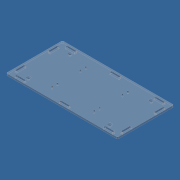
# Autodesk Inventor part: P1704_205
Saved by Autodesk Inventor 2015 (Build 190159000, 159)
## iProperties
Created: 2017-02-08
Part Number: P1704_205
Project: Manette
Material: Plastique PMMA
Description: Socle- Table
Document SubType Name: Modeling
Designer: Alexandre.PICOTTE
Authority: 185x93.4x3
Density: 1.188 g/cm^3
Appearance: Transparent - Clair
Mass: 59.5295 g
Surface Area: 366.091 cm^2
Volume: 50.109 cm^3
Material number: ---
Author: Boris.GAUDARD
Autodesk Inventor part; units mm, degrees
ref_plane "Plan YZ" through (0, 0, 0) normal (1, 0, 0) x (0, 1, 0)
ref_plane "Plan XZ" through (0, 0, 0) normal (0, 1, 0) x (-1, 0, 0)
ref_plane "Plan XY" through (0, 0, 0) normal (0, 0, 1) x (1, 0, 0)
sketch "Esquisse1" plane through (0, 0, 0) normal (0, 0, 1) x (1, 0, 0)
  line L0 (-92.5, 46.7) -> (92.5, 46.7)
  line L1 (92.5, 46.7) -> (92.5, -46.7)
  line L2 (92.5, -46.7) -> (-92.5, -46.7)
  line L3 (-92.5, -46.7) -> (-92.5, 46.7)
  line L4 (0, -65.38) -> (0, 65.38) construction
  line L5 (-129.5, 0) -> (129.5, 0) construction
  point P0 (0, 0)
  dimension "d0" = 185
  dimension "d1" = 93.4
  constraints: 8 end point, 2 parallel, 1 horizontal, 1 perpendicular, 2 other
  measures "d0" distance between parallel lines of L1 L3
  measures "d1" distance between parallel lines of L0 L2
extrude "Extrusion1" add sketch "Esquisse1" along normal blind 3
fillet "Congé1" radius 2 4 edges at (-92.5, 46.7, 1.5) (92.5, 46.7, 1.5) (92.5, -46.7, 1.5) (-92.5, -46.7, 1.5)
sketch "Esquisse21" plane through (0, 0, 3) normal (0, 0, 1) x (1, 0, 0)
  line L0 (-129.5, 0) -> (129.5, 0) construction
  line L1 (0, -85.38) -> (0, 87.38) construction
  line L2 (-7.5, 43.7) -> (7.5, 43.7)
  line L3 (7.5, 43.7) -> (7.5, 40.5)
  line L4 (7.5, 40.5) -> (-7.5, 40.5)
  line L5 (-7.5, 40.5) -> (-7.5, 43.7)
  line L6 (-90.5, 46.7) -> (90.5, 46.7) construction
  line L7 (-81, 43.7) -> (-66, 43.7)
  line L8 (-66, 43.7) -> (-66, 40.5)
  line L9 (-66, 40.5) -> (-81, 40.5)
  line L10 (-81, 40.5) -> (-81, 43.7)
  line L11 (-92.5, -44.7) -> (-92.5, 44.7) construction
  line L12 (66, 43.7) -> (81, 43.7)
  line L13 (81, 43.7) -> (81, 40.5)
  line L14 (81, 40.5) -> (66, 40.5)
  line L15 (66, 40.5) -> (66, 43.7)
  line L16 (-81, -40.5) -> (-66, -40.5)
  line L17 (-66, -40.5) -> (-66, -43.7)
  line L18 (-66, -43.7) -> (-81, -43.7)
  line L19 (-81, -43.7) -> (-81, -40.5)
  line L20 (-7.5, -43.7) -> (7.5, -43.7)
  line L21 (7.5, -43.7) -> (7.5, -40.5)
  line L22 (7.5, -40.5) -> (-7.5, -40.5)
  line L23 (-7.5, -40.5) -> (-7.5, -43.7)
  line L24 (66, -43.7) -> (81, -43.7)
  line L25 (81, -43.7) -> (81, -40.5)
  line L26 (81, -40.5) -> (66, -40.5)
  line L27 (66, -40.5) -> (66, -43.7)
  point P0 (0, 0)
  dimension "d216" = 15
  dimension "d217" = 3.2
  dimension "d218" = 3
  dimension "d221" = 11.5
  constraints: 48 end point, 12 parallel, 8 collinear, 6 horizontal, 6 perpendicular, 4 equal length, 1 point on line, 7 other
  measures "d216" distance of L2.start L2.end
  measures "d217" distance of L2.end L3.end
  measures "d218" distance between parallel lines of L6 L2
  measures "d221" distance between parallel lines of L10 L11
extrude "Extrusion8" cut sketch "Esquisse21" against normal through all
sketch "Esquisse23" plane through (0, 0, 3) normal (0, 0, 1) x (1, 0, 0)
  line L0 (0, -65.38) -> (0, 65.38) construction
  line L1 (-129.5, 0) -> (129.5, 0) construction
  point P0 (0, 0)
  point P1 (-67.5, 34.5)
  point P2 (67.5, 34.5)
  point P3 (67.5, -34.5)
  point P4 (-67.5, -34.5)
  dimension "d238" = 135
  dimension "d239" = 69
  constraints: 2 horizontal alignment, 2 symmetric about line, 2 vertical alignment
  measures "d238" distance of point (67.5, 34.5) point (-67.5, 34.5)
  measures "d239" distance of point (-67.5, -34.5) point (-67.5, 34.5)
hole "Perçage11" at (-67.5, 34.5, 3) at (67.5, 34.5, 3) at (67.5, -34.5, 3) at (-67.5, -34.5, 3) direction (0, 0, -1) diameter 3.4 end through all countersink diameter 6.3 countersink angle 90 clearance for "Vis à tête plate fraisée ISO 2009/7046" size "M3" standard "ISO"
sketch "Esquisse24" plane through (0, 0, 3) normal (0, 0, 1) x (1, 0, 0)
  line L0 (0, -87.38) -> (0, 85.38) construction
  line L1 (-89.5, 35.2) -> (-86.5, 35.2)
  line L2 (-86.5, 35.2) -> (-86.5, 20.2)
  line L3 (-86.5, 20.2) -> (-89.5, 20.2)
  line L4 (-89.5, 20.2) -> (-89.5, 35.2)
  line L5 (-89.5, -20.2) -> (-86.5, -20.2)
  line L6 (-86.5, -20.2) -> (-86.5, -35.2)
  line L7 (-86.5, -35.2) -> (-89.5, -35.2)
  line L8 (-89.5, -35.2) -> (-89.5, -20.2)
  line L9 (89.5, -35.2) -> (86.5, -35.2)
  line L10 (86.5, -35.2) -> (86.5, -20.2)
  line L11 (86.5, -20.2) -> (89.5, -20.2)
  line L12 (89.5, -20.2) -> (89.5, -35.2)
  line L13 (86.5, 35.2) -> (89.5, 35.2)
  line L14 (89.5, 35.2) -> (89.5, 20.2)
  line L15 (89.5, 20.2) -> (86.5, 20.2)
  line L16 (86.5, 20.2) -> (86.5, 35.2)
  line L17 (-92.5, -44.7) -> (-92.5, 44.7) construction
  line L18 (-129.5, 0) -> (129.5, 0) construction
  line L19 (90.5, -46.7) -> (-90.5, -46.7) construction
  point P0 (0, 0)
  dimension "d248" = 15
  dimension "d249" = 3
  dimension "d250" = 3
  dimension "d251" = 11.5
  constraints: 32 end point, 8 parallel, 4 collinear, 4 horizontal, 4 perpendicular, 3 point on line, 6 other
  measures "d248" distance of L7.end L5.start
  measures "d249" distance of L5.start L5.end
  measures "d250" distance between parallel lines of L17 L8
  measures "d251" distance between parallel lines of L7 L19
extrude "Extrusion10" cut sketch "Esquisse24" against normal through all
sketch "Esquisse26" plane through (0, 0, 3) normal (0, 0, 1) x (1, 0, 0)
  line L0 (-89.5, 35.2) -> (-86.5, 35.2) construction
  line L1 (-89.5, 20.2) -> (-89.5, 35.2) construction
  line L2 (-86.5, 35.2) -> (-86.5, 20.2) construction
  line L3 (-86.5, 20.2) -> (-89.5, 20.2) construction
  line L4 (-66, 40.5) -> (-81, 40.5) construction
  line L5 (-81, 40.5) -> (-81, 43.7) construction
  line L6 (-81, 43.7) -> (-66, 43.7) construction
  line L7 (-66, 43.7) -> (-66, 40.5) construction
  line L8 (7.5, 40.5) -> (-7.5, 40.5) construction
  line L9 (-7.5, 40.5) -> (-7.5, 43.7) construction
  line L10 (-7.5, 43.7) -> (7.5, 43.7) construction
  line L11 (7.5, 43.7) -> (7.5, 40.5) construction
  line L12 (81, 40.5) -> (66, 40.5) construction
  line L13 (66, 40.5) -> (66, 43.7) construction
  line L14 (66, 43.7) -> (81, 43.7) construction
  line L15 (81, 43.7) -> (81, 40.5) construction
  line L16 (-89.5, -35.2) -> (-89.5, -20.2) construction
  line L17 (-89.5, -20.2) -> (-86.5, -20.2) construction
  line L18 (-86.5, -20.2) -> (-86.5, -35.2) construction
  line L19 (-86.5, -35.2) -> (-89.5, -35.2) construction
  line L20 (-81, -40.5) -> (-66, -40.5) construction
  line L21 (-81, -43.7) -> (-81, -40.5) construction
  line L22 (-66, -43.7) -> (-81, -43.7) construction
  line L23 (-66, -40.5) -> (-66, -43.7) construction
  line L24 (89.5, -20.2) -> (89.5, -35.2) construction
  line L25 (89.5, -35.2) -> (86.5, -35.2) construction
  line L26 (86.5, -35.2) -> (86.5, -20.2) construction
  line L27 (86.5, -20.2) -> (89.5, -20.2) construction
  line L28 (-89.5, 20.2) -> (-89.5, 35.2) construction
  line L29 (-89.5, 35.2) -> (-86.5, 35.2) construction
  line L30 (-86.5, 35.2) -> (-86.5, 20.2) construction
  line L31 (-86.5, 20.2) -> (-89.5, 20.2) construction
  line L32 (-89.5, -35.2) -> (-89.5, -20.2) construction
  line L33 (-89.5, -20.2) -> (-86.5, -20.2) construction
  line L34 (-86.5, -20.2) -> (-86.5, -35.2) construction
  line L35 (-86.5, -35.2) -> (-89.5, -35.2) construction
  line L36 (86.5, 20.2) -> (86.5, 35.2) construction
  line L37 (86.5, 35.2) -> (89.5, 35.2) construction
  line L38 (89.5, 35.2) -> (89.5, 20.2) construction
  line L39 (89.5, 20.2) -> (86.5, 20.2) construction
  circle A0 centre (67.5, -34.5) radius 3.15 construction
  circle A1 centre (-67.5, 34.5) radius 3.15 construction
  circle A2 centre (67.5, 34.5) radius 3.15 construction
  circle A3 centre (-67.5, -34.5) radius 3.15 construction
  line L40 (7.5, -40.5) -> (7.5, -43.7) construction
  line L41 (7.5, -43.7) -> (-7.5, -43.7) construction
  line L42 (-7.5, -43.7) -> (-7.5, -40.5) construction
  line L43 (-7.5, -40.5) -> (7.5, -40.5) construction
  line L44 (66, 40.5) -> (66, 43.7) construction
  line L45 (66, 43.7) -> (81, 43.7) construction
  line L46 (81, 43.7) -> (81, 40.5) construction
  line L47 (81, 40.5) -> (66, 40.5) construction
  line L48 (-7.5, 40.5) -> (-7.5, 43.7) construction
  line L49 (-7.5, 43.7) -> (7.5, 43.7) construction
  line L50 (7.5, 43.7) -> (7.5, 40.5) construction
  line L51 (7.5, 40.5) -> (-7.5, 40.5) construction
  line L52 (-81, 40.5) -> (-81, 43.7) construction
  line L53 (-81, 43.7) -> (-66, 43.7) construction
  line L54 (-66, 43.7) -> (-66, 40.5) construction
  line L55 (-66, 40.5) -> (-81, 40.5) construction
  line L56 (-81, -43.7) -> (-81, -40.5) construction
  line L57 (-81, -40.5) -> (-66, -40.5) construction
  line L58 (-66, -40.5) -> (-66, -43.7) construction
  line L59 (-66, -43.7) -> (-81, -43.7) construction
  line L60 (81, -40.5) -> (81, -43.7) construction
  line L61 (81, -43.7) -> (66, -43.7) construction
  line L62 (66, -43.7) -> (66, -40.5) construction
  line L63 (66, -40.5) -> (81, -40.5) construction
  arc A4 (-92.5, -44.7) -> (-90.5, -46.7) centre (-90.5, -44.7) ccw construction
  line L64 (90.5, -46.7) -> (-90.5, -46.7) construction
  arc A5 (90.5, -46.7) -> (92.5, -44.7) centre (90.5, -44.7) ccw construction
  line L65 (92.5, 44.7) -> (92.5, -44.7) construction
  arc A6 (92.5, 44.7) -> (90.5, 46.7) centre (90.5, 44.7) ccw construction
  line L66 (-90.5, 46.7) -> (90.5, 46.7) construction
  arc A7 (-90.5, 46.7) -> (-92.5, 44.7) centre (-90.5, 44.7) ccw construction
  line L67 (-92.5, -44.7) -> (-92.5, 44.7) construction
  point P0 (0, 0)
  constraints: 40 coincident
hole "Perçage12" at (-81, 40.5, 3) at (-81, 43.7, 3) at (-66, 40.5, 3) at (-66, 43.7, 3) at (-86.5, 35.2, 3) at (-89.5, 35.2, 3) at (-89.5, 20.2, 3) at (-86.5, 20.2, 3) at (-86.5, -20.2, 3) at (-89.5, -20.2, 3) at (-89.5, -35.2, 3) at (-86.5, -35.2, 3) at (-81, -40.5, 3) at (-81, -43.7, 3) at (-66, -43.7, 3) at (-66, -40.5, 3) at (-7.5, -43.7, 3) at (-7.5, -40.5, 3) at (7.5, -40.5, 3) at (7.5, -43.7, 3) at (66, -43.7, 3) at (66, -40.5, 3) at (81, -40.5, 3) at (81, -43.7, 3) at (86.5, -35.2, 3) at (86.5, -20.2, 3) at (89.5, -20.2, 3) at (89.5, -35.2, 3) at (86.5, 20.2, 3) at (89.5, 20.2, 3) at (86.5, 35.2, 3) at (89.5, 35.2, 3) at (81, 40.5, 3) at (66, 43.7, 3) at (66, 40.5, 3) at (81, 43.7, 3) at (-7.5, 43.7, 3) at (-7.5, 40.5, 3) at (7.5, 40.5, 3) at (7.5, 43.7, 3) direction (0, 0, -1) diameter 1 end through all
sketch "Esquisse27" plane through (0, 0, 3) normal (0, 0, 1) x (1, 0, 0)
  line L0 (90.5, -46.7) -> (-90.5, -46.7) projected
  line L1 (0, -65.38) -> (0, 65.38) construction
  line L2 (-129.5, 0) -> (129.5, 0) construction
  point P0 (0, 0)
  point P1 (35, -18.95)
  point P2 (35, -27.95)
  point P3 (-35, -18.95)
  point P4 (-35, -27.95)
  point P5 (35, 18.95)
  point P6 (35, 27.95)
  point P7 (-35, 18.95)
  point P8 (-35, 27.95)
  dimension "d263" = 9
  dimension "d265" = 37.9
  dimension "d266" = 70
  constraints: 6 symmetric about line, 2 vertical alignment
  measures "d263" distance of point (35, -18.95) point (35, -27.95)
  measures "d265" distance of point (35, 18.95) point (35, -18.95)
  measures "d266" distance of point (-35, 18.95) point (35, 18.95)
hole "Perçage13" at (35, -18.95, 3) at (35, -27.95, 3) at (-35, -18.95, 3) at (-35, -27.95, 3) at (35, 18.95, 3) at (35, 27.95, 3) at (-35, 18.95, 3) at (-35, 27.95, 3) direction (0, 0, -1) diameter 2.013 end through all thread size "M2.5x0.45" class "6H" standard "ISO M"
